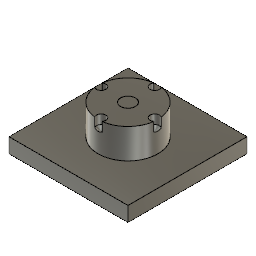
rotating nest on table v4 (Autodesk Fusion 360 design; units mm, degrees)
Autodesk Fusion 360 part; units mm, degrees
sketch "bottom plate" plane through (0, 0, 0) normal (0, 0, 1) x (1, 0, 0)
  line L0 (-20, 20) -> (20, 20)
  line L1 (20, 20) -> (20, -20)
  line L2 (20, -20) -> (-20, -20)
  line L3 (-20, -20) -> (-20, 20)
  line L4 (-20, 20) -> (20, -20) construction
  line L5 (20, 20) -> (-20, -20) construction
  dimension "d1" = 40
  dimension "d2" = 40
  constraint horizontal L0
  constraint perpendicular L0 L1
  constraint parallel L0 L2
  constraint parallel L1 L3
  constraint coincident L4 origin
  constraint coincident L5 origin
  measures "d1" distance of L1.end L2.end
  measures "d2" distance of L0.end L1.end
extrude "Extrude1" add sketch "bottom plate" along normal mid plane 5 makes body 1
sketch "axle" plane through (0, 0, 2.5) normal (0, 0, 1) x (-1, 0, 0)
  line L0 (20, 20) -> (-20, 20)
  line L1 (-20, 20) -> (-20, -20)
  line L2 (-20, -20) -> (20, -20)
  line L3 (20, -20) -> (20, 20)
  line L4 (20, 0) -> (-20, 0) construction
  line L5 (0, -20) -> (0, 20) construction
  circle A0 centre (0, 0) radius 2.5
  dimension "d6" = 5
  constraint midpoint L3 L4.start
  constraint midpoint L1 L4.end
  constraint midpoint L2 L5.start
  constraint midpoint L0 L5.end
  constraint coincident A0.centre origin
  measures "d6" diameter of A0
extrude "Extrude2" add sketch "axle" along normal blind 10 contours A0 bodies 1
sketch "nest wheel" plane through (0, 0, 2.5) normal (0, 0, 1) x (-1, 0, 0) in component "Nest Wheel"
  circle A0 centre (0, 0) radius 2.5
  line L0 (20, 20) -> (-20, 20)
  line L1 (-20, 20) -> (-20, -20)
  line L2 (-20, -20) -> (20, -20)
  line L3 (20, -20) -> (20, 20)
  circle A1 centre (0, 0) radius 10
  line L4 (0.0399, -9.9999) -> (0.0399, 9.9999) construction
  line L5 (10, 0) -> (9.073, 0)
  line L6 (10, 0) -> (-10, 0) construction
  point P0 (0.0399, -9.0727)
  point P1 (9.0727, 0.0399)
  point P2 (-0.0399, 9.0727)
  point P3 (-9.0727, -0.0399)
  dimension "d9" = 20
  dimension "d10" = 19.9998
  dimension "d13" = 360
  dimension "d14" = 9.0727
  constraint coincident A0.centre A1.centre
  constraint coincident A1 L4.start
  constraint coincident A1 L4.end
  constraint vertical L4
  constraint coincident A1 L5.start
  constraint perpendicular L4 L5
  constraint coincident L4 P0
  constraint coincident A1 L6.end
  constraint parallel L5 L6
  measures "d9" diameter of A1
  measures "d10" distance of L4.start L4.end
  measures "d14" vertical distance of A0.centre P0
extrude "Extrude1'" add sketch "nest wheel" along normal blind 10 separate body contours A1 makes body 2 in component "Nest Wheel"
move_body "Move1" bodies 2 to x (1, 0, 0) y (0, 1, 0) z (0, 0, 1) at (0, 0, 24) in component "Nest Wheel"
sketch "hole positions" plane through (0, 0, 36.5) normal (0, 0, 1) x (-1, 0, 0) in component "Nest Wheel"
  circle A0 centre (0, 0) radius 2.5
  circle A1 centre (0, 0) radius 10
  line L0 (0, -10) -> (0, 10) construction
  line L1 (10, 0) -> (-10, 0) construction
  point P0 (-10, 0)
  point P1 (0, -9)
  point P2 (9, 0)
  point P3 (0, 9)
  point P4 (-9, 0)
  dimension "d18" = 9
  dimension "d19" = 9
  dimension "d20" = 9
  constraint coincident A1 L0.start
  constraint coincident A1 L0.end
  constraint vertical L0
  constraint coincident A1 L1.start
  constraint coincident P0 L1.end
  constraint perpendicular L0 L1
  constraint coincident L0 P1
  constraint coincident L1 P2
  constraint coincident L0 P3
  constraint coincident L1 P4
  measures "d18" distance of A0.centre P1
  measures "d19" distance of A0.centre P2
  measures "d20" distance of A0.centre P3
hole "Hole1" at (0, 9, 36.5) at (-9, 0, 36.5) at (9, 0, 36.5) at (0, -9, 36.5) direction (0, 0, -1) diameter 3.1 depth 3.1 tip angle 118 bodies 2 in component "Nest Wheel"
component "Nest Wheel" placed x (1, 0, 0) y (0, 1, 0) z (0, 0, 1) at (0, 0, -24)
named bodies: "Bottom Plate", "nest wheel"
